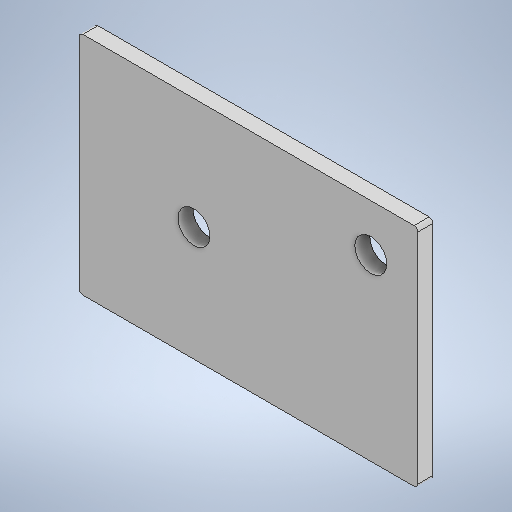
# Autodesk Inventor part: Сrane plate 5
Saved by Autodesk Inventor 2025 (Build 290162010, 162A)
## iProperties
Created: 2024-06-15
Part Number: Сrane plate 5
Material: Generic
Document SubType Name: Sheet Metal
Designer: admin
Density: 1 g/cm^3
Sheet Metal Rule: Default
Appearance: Default
Stock Number: Кран плата 5
Flat Pattern Width: 12 cm
Flat Pattern Length: 18 cm
Flat Pattern Area: 216 cm^2
Sheet Metal Width: 120,000 mm
Sheet Metal Length: 180,000 mm
Sheet Metal Area: 21600,000 mm^2
Author: admin
Autodesk Inventor part; units mm, degrees
ref_plane "YZ Plane" through (0, 0, 0) normal (1, 0, 0) x (0, 1, 0)
ref_plane "XZ Plane" through (0, 0, 0) normal (0, 1, 0) x (-1, 0, 0)
ref_plane "XY Plane" through (0, 0, 0) normal (0, 0, 1) x (1, 0, 0)
sketch "Sketch1" plane through (0, 0, 0) normal (0, 1, 0) x (-1, 0, 0)
  line L0 (90, 60) -> (-90, 60)
  line L1 (-90, 60) -> (-90, -60)
  line L2 (-90, -60) -> (90, -60)
  line L3 (90, -60) -> (90, 60)
  point P0 (0, 0)
  point P1 (0, 60)
  point P2 (90, 0)
  dimension "d0" = 180
  dimension "d1" = 120
  measures "d0" distance of L0.start L0.end
  measures "d1" distance of L2.end L0.start
extrude "Plate1" add sketch "Sketch1" along normal mid plane 8
sketch "Sketch2" plane through (0, -4, 0) normal (0, -1, 0) x (1, 0, 0)
  line L0 (65, 35) -> (-28.9693, 0.798) construction
  line L1 (-90, -60) -> (-90, 60) projected
  line L2 (90, 60) -> (90, -60) projected
  point P0 (0, 0)
  point P1 (-90, 0)
  dimension "d17" = 100
  dimension "d18" = 25
  dimension "d19" = 25
  dimension "d20" = 70
  constraints: 2 end point, 1 coincident, 2 other
  measures "d17" distance of L0.start L0.end
  measures "d18" distance from line of L0.start L2
  measures "d19" horizontal distance of L2.start L0.start
  measures "d20" angle of L2 L0
hole "Hole1" at (65, -4, 35) at (-28.9693, -4, 0.798) direction (0, 1, 0) diameter 17 end through all
fillet "Fillet1" radius 2 4 edges at (90, 0, 60) (-90, 0, 60) (90, 0, -60) (-90, 0, -60)
equation "\"d19\" = d18"
equation "\"d8\" = Thickness"
equation "\"d2\" = Thickness"
equation "\"BendRadius\" = Thickness"
equation "\"BendReliefWidth\" = Thickness"
equation "\"BendReliefDepth\" = 0.5 * Thickness"
equation "\"CornerReliefSize\" = 4 * Thickness"
equation "\"MinimumRemnant\" = 2 * Thickness"
equation "\"TransitionRadius\" = BendRadius"
equation "\"JacobiRadiusSize\" = BendRadius"
equation "\"GapSize\" = Thickness"
equation "\"Thickness\" = 8"
body "Solid1"
